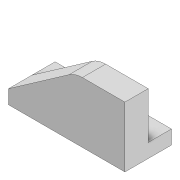
# Autodesk Inventor part: Print_Parts_F1
Saved by Autodesk Inventor 2020 (Build 240168000, 168)
## iProperties
Created: 2020-10-30
Part Number: Print_Parts_F1
Material: Generic
Document SubType Name: Modeling
Designer: magnarecta
Density: 1 g/cm^3
Appearance: Default
Author: magnarecta
Autodesk Inventor part; units mm, degrees
ref_plane "YZ Plane" through (0, 0, 0) normal (1, 0, 0) x (0, 1, 0)
ref_plane "XZ Plane" through (0, 0, 0) normal (0, 1, 0) x (-1, 0, 0)
ref_plane "XY Plane" through (0, 0, 0) normal (0, 0, 1) x (1, 0, 0)
sketch "Sketch1" plane through (0, 0, 0) normal (0, 0, 1) x (1, 0, 0)
  line L0 (0, 0) -> (41.7159, 0)
  line L1 (41.7159, 0) -> (41.7159, 6)
  line L2 (41.7159, 6) -> (0, 6)
  line L3 (0, 6) -> (0, 0)
  line L4 (0, 6) -> (41.7159, 35.2098)
  line L5 (41.7159, 6) -> (41.7159, 35.2098)
  circle A0 centre (31.7159, 16) radius 10
  point P0 (41.7159, 16)
  point P1 (25.9802, 24.1915)
  dimension "d0" = 35
  dimension "d1" = 6
  dimension "d12" = 20
  constraints: 12 end point, 3 tangent, 2 parallel, 1 centre point, 1 collinear, 1 horizontal, 1 perpendicular
  measures "d0" angle of L4 L0
  measures "d1" distance of L0.end L1.end
  measures "d12" diameter of A0
extrude "Extrusion1" add sketch "Sketch1" along normal blind 10 contours L3 L2 L1 L0 | L4 A0 L2 | L2 A0 L5 | A0
sketch "Sketch3" plane through (0, 0, 0) normal (0, 0, -1) x (-1, 0, 0)
  line L0 (-41.7159, 0) -> (-41.7159, 16) projected
  line L1 (0, 0) -> (-41.7159, 0) projected
  line L2 (0, 6) -> (0, 0) projected
  line L3 (-25.9802, 24.1915) -> (0, 6) projected
  line L4 (-47.336, 39.1451) -> (0, 6) projected
  line L5 (-41.7159, 0) -> (0, 0)
  line L6 (0, 0) -> (0, 6)
  line L7 (0, 6) -> (-41.7159, 6)
  line L8 (-41.7159, 6) -> (-41.7159, 0)
  arc A0 (-25.9802, 24.1915) -> (-41.7159, 16) centre (-31.7159, 16) ccw projected
  point P0 (-46.3964, 40.4871)
  constraints: 8 end point, 2 parallel, 1 horizontal, 1 perpendicular
extrude "Extrusion3" add sketch "Sketch3" along normal blind 10 contours L0 L7 L2 L1
sketch "Sketch4" plane through (0, 0, 10) normal (0, 0, 1) x (1, 0, 0)
  line L0 (0, 6) -> (0, 0) projected
  line L1 (0, 0) -> (41.7159, 0) projected
  line L2 (41.7159, 0) -> (41.7159, 16) projected
  arc A0 (41.7159, 16) -> (25.9802, 24.1915) centre (31.7159, 16) ccw projected
  line L3 (25.9802, 24.1915) -> (0, 6) projected
  line L4 (31.7159, 26) -> (50, 26)
  line L5 (50, 26) -> (50, 0)
  line L6 (50, 0) -> (31.7159, 0)
  line L7 (31.7159, 0) -> (31.7159, 26)
  arc A1 (41.7159, 16) -> (25.9802, 24.1915) centre (31.7159, 16) ccw projected
  point P0 (41.7159, 0)
  dimension "d14" = 50
  constraints: 8 end point, 2 parallel, 1 horizontal, 1 perpendicular, 1 tangent, 1 vertical alignment
  measures "d14" distance between parallel lines of L5 L0
extrude "Extrusion4" add sketch "Sketch4" against normal up to surface (10 mm away) contours L4 L5 L6 L2 A0
sketch "Sketch5" plane through (41.7159, 0, 0) normal (1, 0, 0) x (0, 0, -1)
  line L0 (0, 6) -> (0, 0) projected
  line L1 (0, 0) -> (10, 0) projected
  line L2 (10, 6) -> (10, 0) projected
  line L3 (0, 6) -> (10, 6) projected
  point P0 (0, 0)
extrude "Extrusion5" add sketch "Sketch5" along normal up to surface (8.2841 mm away)
body "Solid1"
